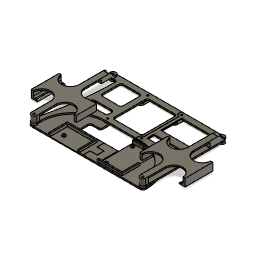
InnerBracket (Autodesk Fusion 360 design; units mm, degrees)
Autodesk Fusion 360 part; units mm, degrees
note: some values were not read from the file. Set by a fixed rule: which face or edge a step refers to.
(part 1 of 2)
sketch "Sketch1" plane through (0, 0, 0) normal (0, 1, 0) x (1, 0, 0) in component "LeftSide"
  line L0 (0, 0) -> (0, -114)
  circle A0 centre (0, 0) radius 1.35
  circle A1 centre (0, -114) radius 1.35
  circle A2 centre (0, -114) radius 4
  circle A3 centre (0, 0) radius 4
  line L1 (0, 0) -> (0, -4)
  line L2 (0, 0) -> (0, 4)
  line L3 (0, 4) -> (10, 4)
  line L4 (10, 4) -> (0, 4)
  line L5 (0, 4) -> (0, -4)
  line L6 (0, -4) -> (10, -4)
  line L7 (10, -4) -> (10, 4)
  line L8 (0, -110) -> (-4, -110)
  line L9 (0, -114) -> (4, -114)
  line L10 (4, -114) -> (-4, -114)
  line L11 (-4, -114) -> (-4, -110)
  line L12 (-4, -110) -> (4, -110)
  line L13 (4, -110) -> (4, -114)
  arc A4 (-4, -110) -> (10, -4) centre (-398.2857, -4) ccw
  line L14 (0, 0) -> (50, 0)
  circle A5 centre (50, 0) radius 1.35
  line L15 (50, 0) -> (99, 0)
  circle A6 centre (99, 0) radius 1.35
  line L16 (99, 0) -> (99, -58)
  line L17 (50, 0) -> (50, -58)
  line L18 (50, -58) -> (99, -58)
  circle A7 centre (99, -58) radius 1.35
  circle A8 centre (50, -58) radius 1.35
  circle A9 centre (50, -58) radius 4
  circle A10 centre (99, -58) radius 4
  circle A11 centre (99, 0) radius 4
  circle A12 centre (50, 0) radius 4
  line L19 (103, 0) -> (103, -58)
  line L20 (99, -62) -> (50, -62)
  line L21 (99, 4) -> (50, 4)
  line L22 (50, 4) -> (10, 4)
  arc A13 (50, -62) -> (4, -110) centre (50, -108.0417) ccw
  dimension "d1" = 114
  dimension "d2" = 2.7
  dimension "d3" = 2.7
  dimension "d4" = 8
  dimension "d5" = 8
  dimension "d6" = 10
  dimension "d7" = 4
  dimension "d8" = 50
  dimension "d9" = 2.7
  dimension "d10" = 49
  dimension "d11" = 2.7
  dimension "d12" = 58
  dimension "d13" = 58
  dimension "d14" = 2.7
  dimension "d15" = 2.7
  dimension "d16" = 8
  dimension "d17" = 8
  dimension "d18" = 8
  dimension "d19" = 8
  constraint coincident L0.start A0.centre
  constraint vertical L0
  constraint coincident L0.end A1.centre
  constraint concentric A1 A2
  constraint concentric A0 A3
  constraint coincident L0 L1.end
  constraint coincident A3 L1.end
  constraint coincident A3 L2.end
  constraint parallel L1 L2
  constraint perpendicular L2 L3
  constraint horizontal L4
  constraint vertical L5
  constraint horizontal L6
  constraint vertical L7
  constraint coincident A2 L8.start
  constraint coincident L0 L8.start
  constraint perpendicular L0 L8
  constraint coincident A2 L9.end
  constraint perpendicular L0 L9
  constraint horizontal L10
  constraint vertical L11
  constraint horizontal L12
  constraint vertical L13
  constraint tangent L7 A4
  constraint perpendicular L0 L14
  constraint coincident L14.end A5.centre
  constraint parallel L14 L15
  constraint coincident L15.end A6.centre
  constraint perpendicular L15 L16
  constraint perpendicular L14 L17
  constraint coincident L16.end L18.end
  constraint coincident L17.end L18.start
  constraint concentric A8 A9
  constraint concentric A7 A10
  constraint concentric A6 A11
  constraint concentric A5 A12
  constraint coincident A11 L19.start
  constraint coincident A10 L19.end
  constraint tangent A10 L19
  constraint vertical L19
  constraint coincident A10 L20.start
  constraint coincident A9 L20.end
  constraint tangent A9 L20
  constraint perpendicular L19 L20
  constraint coincident A11 L21.start
  constraint coincident A12 L21.end
  constraint tangent A12 L21
  constraint parallel L20 L21
  constraint tangent A9 A13
  measures "d1" distance of L0.start L0.end
  measures "d2" diameter of A0
  measures "d3" diameter of A1
  measures "d4" diameter of A2
  measures "d5" diameter of A3
  measures "d6" distance of L2.end L3.end
  measures "d7" distance of L8.start L8.end
  measures "d8" distance of L0.start L14.end
  measures "d9" diameter of A5
  measures "d10" distance of L14.end L15.end
  measures "d11" diameter of A6
  measures "d12" distance of L15.end L16.end
  measures "d13" distance of L14.end L17.end
  measures "d14" diameter of A7
  measures "d15" diameter of A8
  measures "d16" diameter of A9
  measures "d17" diameter of A10
  measures "d18" diameter of A11
  measures "d19" diameter of A12
extrude "Extrude1" add sketch "Sketch1" along normal blind 2 contours L0 A0 A3 L1 L5 L14 | L0 A0 A3 L1 L2 L5 | A0 A3 L2 L5 L14 | A3 L6 L7 L14 | A3 L3 L4 L7 L14 | L0 L7 L12 A4 L14 L17 A9 A12 A13 | L0 L8 L12 A4 | L7 L14 A12 L22 | L0 A1 A2 L9 L10 | A2 L12 L13 | L0 A1 A2 L10 | A2 L8 L11 L12 | L15 A11 A12 L21 | L14 A5 L15 A12 | L14 A5 L17 A12 | A1 A2 L9 L10 | A5 L15 L17 A12 | L15 L16 L17 L18 A9 A10 A11 A12 | L15 A6 L16 A11 | L17 L18 A8 A9 | L18 A9 A10 L20 | L15 A6 L16 A11 | L16 A10 A11 L19 | L17 L18 A8 A9 | L16 L18 A7 A10 | L16 L18 A7 A10 makes body 1 in component "LeftSide"
sketch "Sketch2" plane through (0, 0, 0) normal (0, -1, 0) x (1, 0, 0) in component "LeftSide"
  circle A0 centre (99, 58) radius 1.35
  circle A1 centre (50, 0) radius 1.35
  circle A2 centre (0, 0) radius 1.35
  circle A3 centre (0, 114) radius 1.35
  circle A4 centre (50, 58) radius 1.35
  circle A5 centre (99, 0) radius 1.35
  arc A6 (103, 58) -> (99, 62) centre (99, 58) ccw
  line L0 (99, 62) -> (50, 62)
  arc A7 (4, 110) -> (50, 62) centre (50, 108.0417) ccw
  line L1 (4, 110) -> (4, 114)
  arc A8 (4, 114) -> (-4, 114) centre (0, 114) ccw
  line L2 (-4, 114) -> (-4, 110)
  arc A9 (10, 4) -> (-4, 110) centre (-398.2857, 4) ccw
  line L3 (10, 4) -> (0, 4)
  arc A10 (0, 4) -> (0, -4) centre (0, 0) ccw
  line L4 (0, -4) -> (99, -4)
  arc A11 (99, -4) -> (103, 0) centre (99, 0) ccw
  line L5 (103, 0) -> (103, 58)
  circle A12 centre (0, 0) radius 4
  circle A13 centre (0, 114) radius 4
  circle A14 centre (99, 58) radius 4
  circle A15 centre (50, 58) radius 4
  circle A16 centre (50, 0) radius 4
  circle A17 centre (99, 0) radius 4
  line L6 (50, 0) -> (50, 10)
  line L7 (99, 0) -> (99, 10)
  circle A18 centre (99, 10) radius 4
  circle A19 centre (50, 10) radius 4
  line L8 (95, 10) -> (95, 0)
  line L9 (54, 10) -> (54, 0)
  line L10 (46, 10) -> (46, 0)
  dimension "d404" = 10
  dimension "d405" = 10
  dimension "d406" = 8
  dimension "d407" = 8
  constraint concentric A2 A12
  constraint coincident L3.end A12
  constraint concentric A3 A13
  constraint concentric A0 A14
  constraint coincident A6.end A14
  constraint concentric A4 A15
  constraint coincident L0.end A15
  constraint concentric A1 A16
  constraint tangent L4 A16
  constraint concentric A5 A17
  constraint coincident L4.end A17
  constraint coincident A1.centre A16.centre
  constraint perpendicular L4 L6
  constraint coincident A5.centre A11.centre
  constraint vertical L7
  constraint coincident L7.end A18.centre
  constraint coincident L6.end A19.centre
  constraint coincident A18 L8.start
  constraint coincident A17 L8.end
  constraint tangent A17 L8
  constraint parallel L7 L8
  constraint coincident A19 L9.start
  constraint coincident A16 L9.end
  constraint tangent A16 L9
  constraint parallel L6 L9
  constraint coincident A19 L10.start
  constraint coincident A16 L10.end
  constraint tangent A16 L10
  constraint parallel L6 L10
  measures "d404" distance of A1.centre L6.end
  measures "d405" distance of A5.centre L7.end
  measures "d406" diameter of A18
  measures "d407" diameter of A19
extrude "Extrude2" add sketch "Sketch2" along normal blind 3 contours A6 A14 | A15 | A16 | A18 | L5 A17 L7 A18 | A11 A17 | A17 L7 A18 L8 | A8 A13 | A10 A12 | A16 L6 A19 L10 | A16 L6 A19 L9 | A19 bodies 1 in component "LeftSide"
sketch "Sketch3" plane through (0, 2, 0) normal (0, 1, 0) x (-1, 0, 0) in component "LeftSide"
  circle A0 centre (-99, 58) radius 1.35
  circle A1 centre (-50, 0) radius 1.35
  circle A2 centre (0, 0) radius 1.35
  circle A3 centre (0, 114) radius 1.35
  circle A4 centre (-50, 58) radius 1.35
  circle A5 centre (-99, 0) radius 1.35
  arc A6 (-99, 62) -> (-103, 58) centre (-99, 58) ccw
  line L0 (-103, 58) -> (-103, 0)
  arc A7 (-103, 0) -> (-99, -4) centre (-99, 0) ccw
  line L1 (-99, -4) -> (0, -4)
  arc A8 (0, -4) -> (0, 4) centre (0, 0) ccw
  line L2 (0, 4) -> (-10, 4)
  arc A9 (4, 110) -> (-10, 4) centre (398.2857, 4) ccw
  line L3 (4, 110) -> (4, 114)
  arc A10 (4, 114) -> (-4, 114) centre (0, 114) ccw
  line L4 (-4, 114) -> (-4, 110)
  arc A11 (-50, 62) -> (-4, 110) centre (-50, 108.0417) ccw
  line L5 (-50, 62) -> (-99, 62)
  circle A12 centre (-99, 0) radius 4
  circle A13 centre (-99, 58) radius 4
  line L6 (-95, 58) -> (-95, 62)
  line L7 (-99, 54) -> (-103, 54)
  line L8 (-99, 4) -> (-103, 4)
  line L9 (-95, 0) -> (-95, -4)
  line L10 (-99, 54) -> (-99, 4)
  constraint concentric A5 A12
  constraint coincident A7.end A12
  constraint concentric A0 A13
  constraint coincident A6.start A13
  constraint coincident A13 L6.start
  constraint coincident L5 L6.end
  constraint tangent A13 L6
  constraint perpendicular L5 L6
  constraint coincident A13 L7.start
  constraint coincident L0 L7.end
  constraint tangent A13 L7
  constraint perpendicular L0 L7
  constraint coincident A12 L8.start
  constraint coincident L0 L8.end
  constraint tangent A12 L8
  constraint perpendicular L0 L8
  constraint coincident A12 L9.start
  constraint coincident L1 L9.end
  constraint tangent A12 L9
  constraint perpendicular L1 L9
extrude "Extrude3" cut sketch "Sketch3" against normal blind 1 contours A6 A13 | L5 A13 L6 | L0 A13 L7 | L0 L7 L8 L10 | L0 A12 L8 | A7 A12 | L1 A12 L9 bodies 1 in component "LeftSide"
sketch "Sketch1 (2)" plane through (0, 1, 0) normal (0, 1, 0) x (-1, 0, 0) in component "RightSide"
  circle A0 centre (-99, 58) radius 1.35
  circle A1 centre (-99, 0) radius 1.35
  line L0 (-95, 58) -> (-95, 62)
  line L1 (-95, 62) -> (-99, 62)
  arc A2 (-99, 62) -> (-103, 58) centre (-99, 58) ccw
  line L2 (-103, 58) -> (-103, 0)
  arc A3 (-103, 0) -> (-99, -4) centre (-99, 0) ccw
  line L3 (-99, -4) -> (-95, -4)
  line L4 (-95, -4) -> (-95, 0)
  arc A4 (-95, 0) -> (-99, 4) centre (-99, 0) ccw
  line L5 (-99, 4) -> (-99, 54)
  arc A5 (-99, 54) -> (-95, 58) centre (-99, 58) ccw
  line L6 (-99, 0) -> (-157, 0)
  circle A6 centre (-157, 0) radius 1.35
  circle A7 centre (-157, 0) radius 4
  line L7 (-157, 0) -> (-157, 114)
  circle A8 centre (-157, 114) radius 1.35
  circle A9 centre (-157, 114) radius 4
  line L8 (-161, 114) -> (-161, 0)
  line L9 (-157, -4) -> (-99, -4)
  arc A10 (-153, 114) -> (-99, 62) centre (-100.963, 114) ccw
  dimension "d30" = 58
  dimension "d31" = 2.7
  dimension "d32" = 8
  dimension "d33" = 114
  dimension "d34" = 2.7
  dimension "d35" = 8
  constraint coincident A1.centre A3.centre
  constraint perpendicular L2 L6
  constraint coincident L6.end A6.centre
  constraint concentric A6 A7
  constraint perpendicular L6 L7
  constraint coincident L7.end A8.centre
  constraint concentric A8 A9
  constraint coincident A9 L8.start
  constraint coincident A7 L8.end
  constraint tangent A7 L8
  constraint vertical L8
  constraint coincident A7 L9.start
  constraint coincident A3.end L3.start
  constraint tangent A9 A10
  constraint coincident A9 A10.start
  constraint coincident L1.end A2.start
  measures "d30" distance of A1.centre L6.end
  measures "d31" diameter of A6
  measures "d32" diameter of A7
  measures "d33" distance of L6.end L7.end
  measures "d34" diameter of A8
  measures "d35" diameter of A9
extrude "Extrude1'" add sketch "Sketch1 (2)" along normal blind 1 separate body contours L0 L1 A2 L2 A3 L3 L4 A4 L5 A5 A10 | A2 L2 L6 A7 L7 A9 A10 | A9 | A3 L6 A7 L9 | A7 L7 A9 L8 | L6 A6 A7 L7 | L6 A6 A7 L7 makes body 2 in component "RightSide"
extrude "Extrude2'" add sketch "Sketch1 (2)" against normal blind 1 contours A2 L2 L6 A7 L7 A9 A10 | A9 | A3 L6 A7 L9 | A7 L7 A9 L8 | L6 A6 A7 L7 | L6 A6 A7 L7 bodies 2 in component "RightSide"
sketch "Sketch2 (2)" plane through (0, 0, 0) normal (0, -1, 0) x (1, 0, 0) in component "RightSide"
  circle A0 centre (157, 0) radius 1.35
  circle A1 centre (157, 114) radius 1.35
  line L0 (161, 0) -> (161, 114)
  arc A2 (161, 114) -> (153, 114) centre (157, 114) ccw
  arc A3 (99.2801, 61.9902) -> (153, 114) centre (100.963, 114) ccw
  arc A4 (103, 58) -> (99.2801, 61.9902) centre (99, 58) ccw
  line L1 (103, 58) -> (103, 0)
  arc A5 (99, -4) -> (103, 0) centre (99, 0) ccw
  line L2 (99, -4) -> (157, -4)
  arc A6 (157, -4) -> (161, 0) centre (157, 0) ccw
  circle A7 centre (157, 0) radius 4
  circle A8 centre (157, 114) radius 4
  constraint concentric A0 A7
  constraint coincident L2.end A7
  constraint concentric A1 A8
extrude "Extrude3'" add sketch "Sketch2 (2)" along normal blind 3 contours A6 A7 | A2 A8 bodies 2 in component "RightSide"
sketch "Sketch5" plane through (0, 2, 0) normal (0, 1, 0) x (-1, 0, 0) in component "LeftSide"
  line L0 (-95, 62) -> (-95, 58)
  arc A0 (-99, 54) -> (-95, 58) centre (-99, 58) ccw
  line L1 (-99, 54) -> (-99, 4)
  arc A1 (-95, 0) -> (-99, 4) centre (-99, 0) ccw
  line L2 (-95, 0) -> (-95, -4)
  line L3 (-95, -4) -> (0, -4)
  arc A2 (0, -4) -> (0, 4) centre (0, 0) ccw
  line L4 (0, 4) -> (-10, 4)
  arc A3 (4, 110) -> (-10, 4) centre (398.2857, 4) ccw
  line L5 (4, 110) -> (4, 114)
  arc A4 (4, 114) -> (-4, 114) centre (0, 114) ccw
  line L6 (-4, 114) -> (-4, 110)
  arc A5 (-50, 62) -> (-4, 110) centre (-50, 108.0417) ccw
  line L7 (-50, 62) -> (-95, 62)
  circle A6 centre (0, 114) radius 1.35
  circle A7 centre (0, 0) radius 1.35
  line L8 (-50, 0) -> (-99, 58)
  line L9 (-99, 58) -> (-95.7732, 54.1806)
  line L10 (-50, 0) -> (-53.2268, 3.8194)
  line L11 (-53.2268, 3.8194) -> (-95.7732, 3.8194)
  line L12 (-95.7732, 3.8194) -> (-95.7732, 54.1806)
  line L13 (-95.7732, 54.1806) -> (-53.2268, 54.1806)
  line L14 (-53.2268, 54.1806) -> (-53.2268, 3.8194)
  line L15 (-53.2268, 3.8194) -> (-45.2268, 3.8194)
  line L16 (-45.2268, 3.8194) -> (-15.2268, 3.8194)
  line L17 (-15.2268, 3.8194) -> (-15.2268, 33.8194)
  line L18 (-15.2268, 33.8194) -> (-45.2268, 33.8194)
  line L19 (-45.2268, 33.8194) -> (-45.2268, 3.8194)
  line L20 (-53.2268, 54.1806) -> (-45.2268, 54.1806)
  line L21 (-45.2268, 54.1806) -> (-15.2268, 54.1806)
  line L22 (-15.2268, 54.1806) -> (-15.2268, 44.1806)
  line L23 (-15.2268, 44.1806) -> (-45.2268, 44.1806)
  line L24 (-45.2268, 44.1806) -> (-45.2268, 54.1806)
  circle A8 centre (-50, 58) radius 1.35
  circle A9 centre (-50, 0) radius 1.35
  dimension "d54" = 5
  dimension "d55" = 5
  dimension "d56" = 8
  dimension "d57" = 30
  dimension "d58" = 30
  dimension "d59" = 8
  dimension "d60" = 30
  dimension "d61" = 10
  constraint coincident A0.centre L8.end
  constraint parallel L8 L9
  constraint parallel L8 L10
  constraint horizontal L11
  constraint vertical L12
  constraint horizontal L13
  constraint vertical L14
  constraint perpendicular L14 L15
  constraint horizontal L16
  constraint vertical L17
  constraint horizontal L18
  constraint vertical L19
  constraint perpendicular L14 L20
  constraint horizontal L21
  constraint vertical L22
  constraint horizontal L23
  constraint vertical L24
  measures "d54" distance of A0.centre L9.end
  measures "d55" distance of L8.start L10.end
  measures "d56" distance of L10.end L15.end
  measures "d57" distance of L15.end L16.end
  measures "d58" distance of L15.end L18.end
  measures "d59" distance of L13.end L20.end
  measures "d60" distance of L20.end L21.end
  measures "d61" distance of L20.end L23.end
extrude "Extrude5" cut sketch "Sketch5" against normal blind 2 contours L8 L11 L12 | L8 L13 L14 | L16 L17 L18 L19 | L21 L22 L23 L24 bodies 1 in component "LeftSide"
sketch "Sketch4" plane through (0, 2, 0) normal (0, 1, 0) x (-1, 0, 0) in component "RightSide"
  circle A0 centre (-157, 0) radius 1.35
  circle A1 centre (-157, 114) radius 1.35
  line L0 (-161, 114) -> (-161, 0)
  arc A2 (-161, 0) -> (-157, -4) centre (-157, 0) ccw
  line L1 (-157, -4) -> (-95, -4)
  line L2 (-95, -4) -> (-95, 0)
  arc A3 (-95, 0) -> (-99, 4) centre (-99, 0) ccw
  line L3 (-99, 4) -> (-99, 54)
  arc A4 (-99, 54) -> (-95, 58) centre (-99, 58) ccw
  line L4 (-95, 58) -> (-95, 62)
  line L5 (-95, 62) -> (-99, 62)
  arc A5 (-153, 114) -> (-99, 62) centre (-100.963, 114) ccw
  arc A6 (-153, 114) -> (-161, 114) centre (-157, 114) ccw
  line L6 (-99, 4) -> (-103, 4)
  line L7 (-103, 4) -> (-153, 4)
  line L8 (-153, 4) -> (-153, 34)
  line L9 (-153, 34) -> (-103, 34)
  line L10 (-103, 34) -> (-103, 4)
  line L11 (-99, 54) -> (-103, 54)
  line L12 (-103, 54) -> (-153, 54)
  line L13 (-153, 54) -> (-153, 44)
  line L14 (-153, 44) -> (-103, 44)
  line L15 (-103, 44) -> (-103, 54)
  line L16 (-153, 54) -> (-153, 62)
  line L17 (-153, 62) -> (-152.0608, 62)
  line L18 (-152.0608, 62) -> (-122.0608, 62)
  line L19 (-153, 62) -> (-153, 92)
  arc A7 (-153, 92) -> (-122.0608, 62) centre (-122.9857, 92) ccw
  circle A8 centre (-99, 0) radius 1.35
  circle A9 centre (-99, 58) radius 1.35
  dimension "d64" = 4
  dimension "d65" = 50
  dimension "d66" = 30
  dimension "d67" = 4
  dimension "d68" = 50
  dimension "d69" = 10
  dimension "d105" = 8
  dimension "d106" = 30
  dimension "d107" = 30
  constraint coincident A3.end L3.start
  constraint perpendicular L3 L6
  constraint horizontal L7
  constraint vertical L8
  constraint horizontal L9
  constraint vertical L10
  constraint coincident L3.end A4.start
  constraint perpendicular L3 L11
  constraint horizontal L12
  constraint vertical L13
  constraint horizontal L14
  constraint vertical L15
  constraint perpendicular L12 L16
  constraint perpendicular L16 L17
  constraint perpendicular L16 L18
  constraint perpendicular L17 L19
  constraint tangent L19 A7
  measures "d64" distance of A3.end L6.end
  measures "d65" distance of L6.end L7.end
  measures "d66" distance of L6.end L9.end
  measures "d67" distance of L3.end L11.end
  measures "d68" distance of L11.end L12.end
  measures "d69" distance of L11.end L14.end
  measures "d105" distance of L12.end L16.end
  measures "d106" distance of L17.end L18.end
  measures "d107" distance of L16.end L19.end
extrude "Extrude5'" cut sketch "Sketch4" against normal blind 2 contours L7 L8 L9 L10 | L12 L13 L14 L15 | L17 L18 L19 A7 bodies 2 in component "RightSide"
fillet "Fillet3" radius 3 13 edges at (15.2268, 1, 3.8194) (45.2268, 1, 3.8194) (10, 1, 4) (45.2268, 1, 33.8194) (15.2268, 1, 33.8194) (15.2268, 1, 54.1806) (45.2268, 1, 54.1806) (45.2268, 1, 44.1806) (15.2268, 1, 44.1806) (53.2268, 1, 3.8194) (53.2268, 1, 54.1806) (95.7732, 1, 54.1806) (95.7732, 1, 3.8194) on bodies 1 in component "LeftSide"
fillet "Fillet3'" radius 3 5 edges at (153, 1, 4) (153, 1, 34) (153, 1, 54) (153, 1, 44) (153, 1, 62) on bodies 2 in component "RightSide"
fillet "Fillet4" radius 1 2 edges at (123.9107, 1, 62) (153, 1, 92) on bodies 2 in component "RightSide"
move_face "OffsetFaces1" offset -0.2 5 faces at (98.8097, 1.3333, 3.9955) (95, 1.6667, -1.3333) (99, 1.3333, 37.3333) (98.8097, 1.6667, 54.0045) (95, 1.6667, 59.3333) on bodies 1 in component "LeftSide"
sketch "Sketch1 (3)" plane through (0, 2, 0) normal (0, 1, 0) x (-1, 0, 0) in component "LeftBatteryMount"
  line L0 (-18.2268, 3.8194) -> (-42.2268, 3.8194)
  arc A0 (-45.2268, 6.8194) -> (-42.2268, 3.8194) centre (-42.2268, 6.8194) ccw
  line L1 (-45.2268, 6.8194) -> (-45.2268, 30.8194)
  arc A1 (-42.2268, 33.8194) -> (-45.2268, 30.8194) centre (-42.2268, 30.8194) ccw
  line L2 (-42.2268, 33.8194) -> (-18.2268, 33.8194)
  arc A2 (-15.2268, 30.8194) -> (-18.2268, 33.8194) centre (-18.2268, 30.8194) ccw
  line L3 (-15.2268, 30.8194) -> (-15.2268, 6.8194)
  arc A3 (-18.2268, 3.8194) -> (-15.2268, 6.8194) centre (-18.2268, 6.8194) ccw
  line L4 (-15.2268, 51.1806) -> (-15.2268, 47.1806)
  arc A4 (-18.2268, 44.1806) -> (-15.2268, 47.1806) centre (-18.2268, 47.1806) ccw
  line L5 (-18.2268, 44.1806) -> (-42.2268, 44.1806)
  arc A5 (-45.2268, 47.1806) -> (-42.2268, 44.1806) centre (-42.2268, 47.1806) ccw
  line L6 (-45.2268, 47.1806) -> (-45.2268, 51.1806)
  arc A6 (-42.2268, 54.1806) -> (-45.2268, 51.1806) centre (-42.2268, 51.1806) ccw
  line L7 (-42.2268, 54.1806) -> (-18.2268, 54.1806)
  arc A7 (-15.2268, 51.1806) -> (-18.2268, 54.1806) centre (-18.2268, 51.1806) ccw
  line L8 (-95.7732, 6.8194) -> (-95.7732, 51.1806)
  arc A8 (-92.7732, 54.1806) -> (-95.7732, 51.1806) centre (-92.7732, 51.1806) ccw
  line L9 (-92.7732, 54.1806) -> (-56.2268, 54.1806)
  arc A9 (-53.2268, 51.1806) -> (-56.2268, 54.1806) centre (-56.2268, 51.1806) ccw
  line L10 (-53.2268, 51.1806) -> (-53.2268, 6.8194)
  arc A10 (-56.2268, 3.8194) -> (-53.2268, 6.8194) centre (-56.2268, 6.8194) ccw
  line L11 (-56.2268, 3.8194) -> (-92.7732, 3.8194)
  arc A11 (-95.7732, 6.8194) -> (-92.7732, 3.8194) centre (-92.7732, 6.8194) ccw
  line L12 (-94.8, 62) -> (-94.8, 58)
  arc A12 (-98.8, 53.8048) -> (-94.8, 58) centre (-99, 58) ccw
  line L13 (-98.8, 53.8048) -> (-98.8, 4.1952)
  arc A13 (-94.8, 0) -> (-98.8, 4.1952) centre (-99, 0) ccw
  line L14 (-94.8, 0) -> (-94.8, -4)
  line L15 (-94.8, -4) -> (0, -4)
  arc A14 (0, -4) -> (0, 4) centre (0, 0) ccw
  line L16 (0, 4) -> (-6.9889, 4)
  arc A15 (-9.9888, 7.0222) -> (-6.9889, 4) centre (-6.9889, 7) ccw
  arc A16 (4, 110) -> (-9.9888, 7.0222) centre (398.2857, 4) ccw
  line L17 (4, 110) -> (4, 114)
  arc A17 (4, 114) -> (-4, 114) centre (0, 114) ccw
  line L18 (-4, 114) -> (-4, 110)
  arc A18 (-50, 62) -> (-4, 110) centre (-50, 108.0417) ccw
  line L19 (-50, 62) -> (-94.8, 62)
  circle A19 centre (-50, 58) radius 1.35
  circle A20 centre (0, 114) radius 1.35
  circle A21 centre (0, 0) radius 1.35
  circle A22 centre (-50, 0) radius 1.35
  circle A23 centre (0, 114) radius 4
  line L20 (0, 110) -> (4, 110)
  line L21 (0, 110) -> (-4, 110)
  circle A24 centre (0, 0) radius 4
  line L22 (-4, 110) -> (-4, 21)
  line L23 (-4, 21) -> (4, 21)
  line L24 (4, 21) -> (4, 0)
  line L25 (4, 0) -> (-4, 0)
  line L26 (-4, 0) -> (-4, 21)
  dimension "d154" = 8
  dimension "d155" = 8
  dimension "d156" = 89
  constraint concentric A17 A23
  constraint coincident A23 L20.start
  constraint coincident A16.start L17.start
  constraint tangent A23 L20
  constraint coincident L18.end A18.end
  constraint concentric A14 A24
  constraint perpendicular L21 L22
  constraint horizontal L23
  constraint vertical L24
  constraint horizontal L25
  constraint vertical L26
  constraint midpoint A14 L24.end
  measures "d154" diameter of A23
  measures "d155" diameter of A24
  measures "d156" distance of L18.end L22.end
extrude "Extrude1''" add sketch "Sketch1 (3)" along normal blind 2 separate body contours L18 A23 L21 | A17 A23 | L17 A23 L20 | A14 L16 A24 L23 L24 L26 | L16 A24 L26 | A14 A21 A24 L25 | A14 A21 A24 L25 makes body 3 at (-0.0336, 2, 110.8846) makes body 4 at (0.0336, 2, 14.4487) in component "LeftBatteryMount"
sketch "Sketch2 (3)" plane through (0, 4, 0) normal (0, 1, 0) x (-1, 0, 0) in component "LeftBatteryMount"
  circle A0 centre (0, 0) radius 1.35
  arc A1 (-4, 0) -> (4, 0) centre (0, 0) ccw
  line L0 (4, 0) -> (4, 21)
  line L1 (4, 21) -> (-4, 21)
  line L2 (-4, 21) -> (-4, 0)
  line L3 (-4, 21) -> (4, 21)
  line L4 (4, 21) -> (4, 5)
  line L5 (4, 5) -> (-4, 5)
  line L6 (-4, 5) -> (-4, 21)
  dimension "d159" = 16
  constraint horizontal L3
  constraint vertical L4
  constraint horizontal L5
  constraint vertical L6
  constraint coincident L1.end L2.start
  measures "d159" distance of L1.end L5.end
extrude "Extrude2''" add sketch "Sketch2 (3)" 1 faces at (-0.0336, 4, 110.8846) along normal blind 5 contours L0 L1 L2 L3 L4 L5 L6 on bodies 3 bodies 3 4 in component "LeftBatteryMount"
sketch "Sketch3 (2)" plane through (0, 9, 0) normal (0, 1, 0) x (-1, 0, 0) in component "LeftBatteryMount"
  line L0 (-4, 5) -> (4, 5)
  line L1 (4, 5) -> (4, 21)
  line L2 (4, 21) -> (-4, 21)
  line L3 (-4, 21) -> (-4, 5)
  line L4 (-4, 21) -> (4, 21)
  line L5 (4, 21) -> (4, 110)
  line L6 (4, 110) -> (-4, 110)
  line L7 (-4, 110) -> (-4, 21)
  dimension "d162" = 8
  dimension "d163" = 89
  constraint horizontal L4
  constraint vertical L5
  constraint horizontal L6
  constraint vertical L7
  constraint coincident L2.end L3.start
  measures "d162" distance of L2.end L1.end
  measures "d163" distance of L2.end L6.end
extrude "Extrude3''" add sketch "Sketch3 (2)" 1 faces at (-0.0336, 9, 110.8846) along normal blind 2 on bodies 3 bodies 3 4 in component "LeftBatteryMount"
sketch "Sketch4 (2)" plane through (0, 9, 0) normal (0, -1, 0) x (1, 0, 0) in component "LeftBatteryMount"
  line L0 (4, 110) -> (-4, 110)
  line L1 (-4, 110) -> (-4, 21)
  line L2 (-4, 21) -> (4, 21)
  line L3 (4, 21) -> (4, 110)
  line L4 (-4, 65.5) -> (-29.5, 65.5)
  line L5 (4, 65.5) -> (29.5, 65.5)
  line L6 (-29.5, 65.5) -> (-29.5, 85.5)
  line L7 (-29.5, 85.5) -> (-32.5, 85.5)
  line L8 (-32.5, 85.5) -> (-32.5, 45.5)
  line L9 (-32.5, 45.5) -> (-29.5, 45.5)
  line L10 (-29.5, 45.5) -> (-29.5, 85.5)
  line L11 (29.5, 65.5) -> (29.5, 85.5)
  line L12 (29.5, 85.5) -> (32.5, 85.5)
  line L13 (32.5, 85.5) -> (32.5, 45.5)
  line L14 (32.5, 45.5) -> (29.5, 45.5)
  line L15 (29.5, 45.5) -> (29.5, 85.5)
  line L16 (-16.75, 65.5) -> (-16.75, 73.5)
  line L17 (-16.75, 65.5) -> (-16.75, 57.5)
  line L18 (16.75, 65.5) -> (16.75, 73.5)
  line L19 (16.75, 65.5) -> (16.75, 57.5)
  arc A0 (-29.5, 85.5) -> (-4, 85.2119) centre (-16.7395, 86.2846) ccw
  arc A1 (-4, 45.5) -> (-29.5, 45.5) centre (-16.75, 44.7266) ccw
  arc A2 (29.5, 45.5) -> (4, 45.5) centre (16.75, 44.7266) ccw
  arc A3 (4, 85.5) -> (29.5, 85.5) centre (16.75, 86.2734) ccw
  dimension "d166" = 25.5
  dimension "d167" = 25.5
  dimension "d168" = 20
  dimension "d169" = 3
  dimension "d170" = 40
  dimension "d171" = 20
  dimension "d172" = 3
  dimension "d173" = 40
  dimension "d174" = 8
  dimension "d175" = 8
  dimension "d176" = 8
  dimension "d177" = 8
  constraint midpoint L1 L4.start
  constraint perpendicular L1 L4
  constraint midpoint L3 L5.start
  constraint perpendicular L3 L5
  constraint perpendicular L4 L6
  constraint horizontal L7
  constraint vertical L8
  constraint horizontal L9
  constraint vertical L10
  constraint perpendicular L5 L11
  constraint horizontal L12
  constraint vertical L13
  constraint horizontal L14
  constraint vertical L15
  constraint midpoint L4 L16.start
  constraint perpendicular L4 L16
  constraint perpendicular L4 L17
  constraint midpoint L5 L18.start
  constraint perpendicular L5 L18
  constraint perpendicular L5 L19
  constraint coincident L16.end A0
  constraint coincident L1 A0.end
  constraint coincident L17.end A1
  constraint coincident L1 A1.start
  constraint coincident L19.end A2
  constraint coincident L3 A2.end
  constraint coincident L18.end A3
  constraint coincident L3 A3.start
  measures "d166" distance of L4.start L4.end
  measures "d167" distance of L5.start L5.end
  measures "d168" distance of L4.end L6.end
  measures "d169" distance of L6.end L7.end
  measures "d170" distance of L6.end L9.end
  measures "d171" distance of L5.end L11.end
  measures "d172" distance of L11.end L12.end
  measures "d173" distance of L11.end L14.end
  measures "d174" distance of L16.start L16.end
  measures "d175" distance of L16.start L17.end
  measures "d176" distance of L18.start L18.end
  measures "d177" distance of L18.start L19.end
extrude "Extrude4" add sketch "Sketch4 (2)" against normal blind 2 contours L3 L5 L18 A3 | L1 L4 L16 A0 | L3 L5 L19 A2 | L5 L11 L15 L18 A3 | L1 L4 L17 A1 | L4 L6 L10 L16 A0 | L5 L15 L19 A2 | L11 L12 L13 L14 L15 | L4 L10 L17 A1 | L6 L7 L8 L9 L10 bodies 3 in component "LeftBatteryMount"
sketch "Sketch5 (2)" plane through (0, 9, 0) normal (0, -1, 0) x (1, 0, 0) in component "LeftBatteryMount"
  line L0 (4, 110) -> (-4, 110)
  line L1 (-4, 110) -> (-4, 85.2119)
  arc A0 (-29.5, 85.5) -> (-4, 85.2119) centre (-16.7395, 86.2846) ccw
  line L2 (-29.5, 85.5) -> (-32.5, 85.5)
  line L3 (-32.5, 85.5) -> (-32.5, 45.5)
  line L4 (-32.5, 45.5) -> (-29.5, 45.5)
  arc A1 (-4, 45.5) -> (-29.5, 45.5) centre (-16.75, 44.7266) ccw
  line L5 (-4, 45.5) -> (-4, 21)
  line L6 (-4, 21) -> (4, 21)
  line L7 (4, 21) -> (4, 45.5)
  arc A2 (29.5, 45.5) -> (4, 45.5) centre (16.75, 44.7266) ccw
  line L8 (29.5, 45.5) -> (32.5, 45.5)
  line L9 (32.5, 45.5) -> (32.5, 85.5)
  line L10 (32.5, 85.5) -> (29.5, 85.5)
  arc A3 (4, 85.5) -> (29.5, 85.5) centre (16.75, 86.2734) ccw
  line L11 (4, 85.5) -> (4, 110)
  line L12 (-29.5, 85.5) -> (-29.5, 45.5)
  line L13 (29.5, 85.5) -> (29.5, 45.5)
  constraint coincident A0.start L2.start
  constraint coincident L4.end A1.end
  constraint coincident L10.end A3.end
  constraint coincident A2.start L8.start
extrude "Extrude5''" add sketch "Sketch5 (2)" along normal blind 7 contours L8 L9 L10 L13 | L2 L3 L4 L12 bodies 3 in component "LeftBatteryMount"
sketch "Sketch6" plane through (0, 2, 0) normal (0, -1, 0) x (1, 0, 0) in component "LeftBatteryMount"
  line L0 (-32.5, 85.5) -> (-32.5, 45.5)
  line L1 (-32.5, 45.5) -> (-29.5, 45.5)
  line L2 (-29.5, 45.5) -> (-29.5, 85.5)
  line L3 (-29.5, 85.5) -> (-32.5, 85.5)
  line L4 (-29.5, 85.5) -> (-23.5, 85.5)
  line L5 (-23.5, 85.5) -> (-23.5, 45.5)
  line L6 (-23.5, 45.5) -> (-29.5, 45.5)
  line L7 (-29.5, 45.5) -> (-29.5, 85.5)
  dimension "d182" = 6
  dimension "d183" = 40
  constraint horizontal L4
  constraint vertical L5
  constraint horizontal L6
  constraint vertical L7
  constraint coincident L2.end L3.start
  measures "d182" distance of L2.end L4.end
  measures "d183" distance of L2.end L1.end
extrude "Extrude6" add sketch "Sketch6" along normal blind 2 bodies 3 in component "LeftBatteryMount"
fillet "Fillet1" radius 5 2 edges at (0, 11, 5) (0, 4, 5) on bodies 3 in component "LeftBatteryMount"
fillet "Fillet2" radius 2 2 edges at (-29.5, 2, 65.5) (-23.5, 2, 65.5) on bodies 3 in component "LeftBatteryMount"
sketch "Sketch1 (4)" plane through (0, 2, 0) normal (0, 1, 0) x (-1, 0, 0) in component "RightBatteryMount"
  line L0 (-153, 7) -> (-153, 31)
  arc A0 (-150, 34) -> (-153, 31) centre (-150, 31) ccw
  line L1 (-150, 34) -> (-103, 34)
  line L2 (-103, 34) -> (-103, 4)
  line L3 (-103, 4) -> (-150, 4)
  arc A1 (-153, 7) -> (-150, 4) centre (-150, 7) ccw
  line L4 (-150, 54) -> (-103, 54)
  line L5 (-103, 54) -> (-103, 44)
  line L6 (-103, 44) -> (-150, 44)
  arc A2 (-153, 47) -> (-150, 44) centre (-150, 47) ccw
  line L7 (-153, 47) -> (-153, 51)
  arc A3 (-150, 54) -> (-153, 51) centre (-150, 51) ccw
  arc A4 (-151.0645, 81.3962) -> (-133.626, 63.9351) centre (-122.9857, 92) ccw
  arc A5 (-133.9805, 62) -> (-133.626, 63.9351) centre (-133.9805, 63) ccw
  line L8 (-133.9805, 62) -> (-150, 62)
  arc A6 (-153, 65) -> (-150, 62) centre (-150, 65) ccw
  line L9 (-153, 65) -> (-153, 81.0429)
  arc A7 (-151.0645, 81.3962) -> (-153, 81.0429) centre (-152, 81.0429) ccw
  circle A8 centre (-157, 0) radius 1.35
  circle A9 centre (-99, 58) radius 1.35
  circle A10 centre (-157, 114) radius 1.35
  circle A11 centre (-99, 0) radius 1.35
  line L10 (-161, 114) -> (-161, 0)
  arc A12 (-161, 0) -> (-157, -4) centre (-157, 0) ccw
  line L11 (-157, -4) -> (-95, -4)
  line L12 (-95, -4) -> (-95, 0)
  arc A13 (-95, 0) -> (-99, 4) centre (-99, 0) ccw
  line L13 (-99, 4) -> (-99, 54)
  arc A14 (-99, 54) -> (-95, 58) centre (-99, 58) ccw
  line L14 (-95, 58) -> (-95, 62)
  line L15 (-95, 62) -> (-99, 62)
  arc A15 (-153, 114) -> (-99, 62) centre (-100.963, 114) ccw
  arc A16 (-153, 114) -> (-161, 114) centre (-157, 114) ccw
  circle A17 centre (-157, 0) radius 4
  circle A18 centre (-157, 114) radius 4
  line L16 (-157, 114) -> (-157, 110)
  line L17 (-153, 114) -> (-153, 110)
  line L18 (-153, 110) -> (-161, 110)
  line L19 (-161, 110) -> (-161, 21)
  line L20 (-161, 21) -> (-153, 21)
  line L21 (-153, 21) -> (-153, 0)
  line L22 (-153, 0) -> (-161, 0)
  line L23 (-161, 0) -> (-161, 21)
  dimension "d190" = 8
  dimension "d191" = 8
  dimension "d192" = 89
  constraint concentric A8 A17
  constraint concentric A10 A18
  constraint coincident A10.centre A16.centre
  constraint coincident A18 L16.end
  constraint vertical L16
  constraint coincident A15.start A16.start
  constraint tangent A15 L17
  constraint coincident L10 L18.end
  constraint perpendicular L10 L18
  constraint perpendicular L18 L19
  constraint horizontal L20
  constraint vertical L21
  constraint horizontal L22
  constraint vertical L23
  constraint coincident A17 L21.end
  measures "d190" diameter of A17
  measures "d191" diameter of A18
  measures "d192" distance of L18.end L19.end
extrude "Extrude1'''" add sketch "Sketch1 (4)" along normal blind 2 separate body contours L0 L10 A17 L20 L21 L23 | A8 A17 L22 | A8 A12 A17 L22 | L10 A18 L18 | A16 A18 | A18 L17 L18 makes body 5 at (157.0336, 2, 14.4487) makes body 6 at (157.0336, 2, 110.8846) in component "RightBatteryMount"
sketch "Sketch2 (4)" plane through (0, 4, 0) normal (0, 1, 0) x (-1, 0, 0) in component "RightBatteryMount"
  circle A0 centre (-157, 0) radius 1.35
  arc A1 (-161, 0) -> (-153, 0) centre (-157, 0) ccw
  line L0 (-153, 0) -> (-153, 21)
  line L1 (-153, 21) -> (-161, 21)
  line L2 (-161, 21) -> (-161, 0)
  line L3 (-161, 21) -> (-153, 21)
  line L4 (-153, 21) -> (-153, 5)
  line L5 (-153, 5) -> (-161, 5)
  line L6 (-161, 5) -> (-161, 21)
  dimension "d195" = 16
  constraint horizontal L3
  constraint vertical L4
  constraint horizontal L5
  constraint vertical L6
  constraint coincident L1.end L2.start
  measures "d195" distance of L1.end L5.end
extrude "Extrude2'''" add sketch "Sketch2 (4)" 1 faces at (157.0336, 4, 110.8846) along normal blind 5 contours L0 L1 L2 L3 L4 L5 L6 on bodies 6 bodies 6 5 in component "RightBatteryMount"
sketch "Sketch3 (3)" plane through (0, 9, 0) normal (0, 1, 0) x (-1, 0, 0) in component "RightBatteryMount"
  line L0 (-161, 5) -> (-153, 5)
  line L1 (-153, 5) -> (-153, 21)
  line L2 (-153, 21) -> (-161, 21)
  line L3 (-161, 21) -> (-161, 5)
  line L4 (-161, 21) -> (-161, 110)
  line L5 (-161, 110) -> (-153, 110)
  line L6 (-153, 110) -> (-153, 21)
  line L7 (-153, 21) -> (-161, 21)
  line L8 (-161, 21) -> (-161, 110)
  dimension "d198" = 89
  constraint coincident L2.end L3.start
  constraint perpendicular L2 L4
  constraint horizontal L5
  constraint vertical L6
  constraint horizontal L7
  constraint vertical L8
  constraint coincident L1.end L2.start
  measures "d198" distance of L2.end L4.end
extrude "Extrude3'''" add sketch "Sketch3 (3)" 1 faces at (157.0336, 9, 110.8846) along normal blind 2 on bodies 6 bodies 6 5 in component "RightBatteryMount"
sketch "Sketch4 (3)" plane through (0, 9, 0) normal (0, -1, 0) x (1, 0, 0) in component "RightBatteryMount"
  line L0 (161, 110) -> (153, 110)
  line L1 (153, 110) -> (153, 21)
  line L2 (153, 21) -> (161, 21)
  line L3 (161, 21) -> (161, 110)
  line L4 (161, 65.5) -> (186.5, 65.5)
  line L5 (153, 65.5) -> (127.5, 65.5)
  line L6 (127.5, 65.5) -> (127.5, 85.5)
  line L7 (186.5, 65.5) -> (186.5, 85.5)
  line L8 (186.5, 85.5) -> (189.5, 85.5)
  line L9 (189.5, 85.5) -> (189.5, 45.5)
  line L10 (189.5, 45.5) -> (186.5, 45.5)
  line L11 (186.5, 45.5) -> (186.5, 85.5)
  line L12 (127.5, 85.5) -> (124.5, 85.5)
  line L13 (124.5, 85.5) -> (124.5, 45.5)
  line L14 (124.5, 45.5) -> (127.5, 45.5)
  line L15 (127.5, 45.5) -> (127.5, 85.5)
  line L16 (140.25, 65.5) -> (140.25, 57.5)
  line L17 (140.25, 65.5) -> (140.25, 73.5)
  line L18 (173.75, 65.5) -> (173.75, 73.5)
  line L19 (173.75, 65.5) -> (173.75, 57.5)
  arc A0 (127.5, 85.5) -> (153, 85.5) centre (140.25, 86.2734) ccw
  arc A1 (161, 85.5) -> (186.5, 85.5) centre (173.75, 86.2734) ccw
  arc A2 (186.5, 45.5) -> (161, 45.5) centre (173.75, 44.7266) ccw
  arc A3 (153, 45.5) -> (127.5, 45.5) centre (140.25, 44.7266) ccw
  dimension "d201" = 25.5
  dimension "d202" = 25.5
  dimension "d203" = 20
  dimension "d204" = 20
  dimension "d205" = 3
  dimension "d206" = 40
  dimension "d207" = 3
  dimension "d208" = 40
  dimension "d209" = 8
  dimension "d210" = 8
  dimension "d211" = 8
  dimension "d212" = 8
  constraint midpoint L3 L4.start
  constraint perpendicular L3 L4
  constraint midpoint L1 L5.start
  constraint perpendicular L1 L5
  constraint perpendicular L5 L6
  constraint perpendicular L4 L7
  constraint horizontal L8
  constraint vertical L9
  constraint horizontal L10
  constraint vertical L11
  constraint horizontal L12
  constraint vertical L13
  constraint horizontal L14
  constraint vertical L15
  constraint midpoint L5 L16.start
  constraint perpendicular L5 L16
  constraint perpendicular L5 L17
  constraint midpoint L4 L18.start
  constraint perpendicular L4 L18
  constraint perpendicular L4 L19
  constraint coincident L17.end A0
  constraint coincident L1 A0.end
  constraint coincident L18.end A1
  constraint coincident L3 A1.start
  constraint coincident L19.end A2
  constraint coincident L3 A2.end
  constraint coincident L16.end A3
  constraint coincident L1 A3.start
  measures "d201" distance of L4.start L4.end
  measures "d202" distance of L5.start L5.end
  measures "d203" distance of L5.end L6.end
  measures "d204" distance of L4.end L7.end
  measures "d205" distance of L7.end L8.end
  measures "d206" distance of L7.end L10.end
  measures "d207" distance of L6.end L12.end
  measures "d208" distance of L6.end L14.end
  measures "d209" distance of L16.start L16.end
  measures "d210" distance of L16.start L17.end
  measures "d211" distance of L18.start L18.end
  measures "d212" distance of L18.start L19.end
extrude "Extrude4'" add sketch "Sketch4 (3)" against normal blind 2 contours L3 L4 L18 A1 | L1 L5 L17 A0 | L3 L4 L19 A2 | L4 L7 L11 L18 A1 | L1 L5 L16 A3 | L5 L6 L15 L17 A0 | L4 L11 L19 A2 | L7 L8 L9 L10 L11 | L5 L15 L16 A3 | L6 L12 L13 L14 L15 bodies 6 in component "RightBatteryMount"
sketch "Sketch5 (3)" plane through (0, 9, 0) normal (0, -1, 0) x (1, 0, 0) in component "RightBatteryMount"
  line L0 (161, 110) -> (153, 110)
  line L1 (153, 110) -> (153, 85.5)
  arc A0 (127.5, 85.5) -> (153, 85.5) centre (140.25, 86.2734) ccw
  line L2 (127.5, 85.5) -> (124.5, 85.5)
  line L3 (124.5, 85.5) -> (124.5, 45.5)
  line L4 (124.5, 45.5) -> (127.5, 45.5)
  arc A1 (153, 45.5) -> (127.5, 45.5) centre (140.25, 44.7266) ccw
  line L5 (153, 45.5) -> (153, 21)
  line L6 (153, 21) -> (161, 21)
  line L7 (161, 21) -> (161, 45.5)
  arc A2 (186.5, 45.5) -> (161, 45.5) centre (173.75, 44.7266) ccw
  line L8 (186.5, 45.5) -> (189.5, 45.5)
  line L9 (189.5, 45.5) -> (189.5, 85.5)
  line L10 (189.5, 85.5) -> (186.5, 85.5)
  arc A3 (161, 85.5) -> (186.5, 85.5) centre (173.75, 86.2734) ccw
  line L11 (161, 85.5) -> (161, 110)
  line L12 (127.5, 85.5) -> (127.5, 45.5)
  line L13 (186.5, 85.5) -> (186.5, 45.5)
  constraint coincident A0.start L2.start
  constraint coincident L4.end A1.end
  constraint coincident L10.end A3.end
  constraint coincident A2.start L8.start
extrude "Extrude5'''" add sketch "Sketch5 (3)" along normal blind 7 contours L8 L9 L10 L13 | L2 L3 L4 L12 bodies 6 in component "RightBatteryMount"
sketch "Sketch6 (2)" plane through (0, 2, 0) normal (0, -1, 0) x (1, 0, 0) in component "RightBatteryMount"
  line L0 (186.5, 85.5) -> (186.5, 45.5)
  line L1 (186.5, 45.5) -> (189.5, 45.5)
  line L2 (189.5, 45.5) -> (189.5, 85.5)
  line L3 (189.5, 85.5) -> (186.5, 85.5)
  line L4 (186.5, 85.5) -> (180.5, 85.5)
  line L5 (180.5, 85.5) -> (180.5, 45.5)
  line L6 (180.5, 45.5) -> (186.5, 45.5)
  line L7 (186.5, 45.5) -> (186.5, 85.5)
  dimension "d217" = 6
  dimension "d218" = 40
  constraint horizontal L4
  constraint vertical L5
  constraint horizontal L6
  constraint vertical L7
  constraint coincident L0.start L3.end
  measures "d217" distance of L0.start L4.end
  measures "d218" distance of L0.start L0.end
extrude "Extrude6'" add sketch "Sketch6 (2)" along normal blind 2 bodies 6 in component "RightBatteryMount"
fillet "Fillet1'" radius 5 2 edges at (157, 11, 5) (157, 4, 5) on bodies 6 in component "RightBatteryMount"
fillet "Fillet2'" radius 2 2 edges at (186.5, 2, 65.5) (180.5, 2, 65.5) on bodies 6 in component "RightBatteryMount"
sketch "Sketch7" plane through (0, 2, 0) normal (0, -1, 0) x (1, 0, 0) in component "LeftBatteryMount"
  circle A0 centre (0, 0) radius 1.35
  arc A1 (-4, 0) -> (4, 0) centre (0, 0) ccw
  line L0 (4, 0) -> (4, 21)
  line L1 (4, 21) -> (-4, 21)
  line L2 (-4, 21) -> (-4, 0)
  line L3 (4, 21) -> (-4, 21)
  line L4 (-4, 21) -> (-4, 6)
  line L5 (-4, 6) -> (4, 6)
  line L6 (4, 6) -> (4, 21)
  dimension "d225" = 15
  constraint horizontal L3
  constraint vertical L4
  constraint horizontal L5
  constraint vertical L6
  constraint coincident L0.end L1.start
  measures "d225" distance of L0.end L5.end
extrude "Extrude7" cut sketch "Sketch7" against normal blind 2 contours L0 L1 L2 L3 L4 L5 L6 bodies 3 in component "LeftBatteryMount"
sketch "Sketch8" plane through (0, 11, 0) normal (0, 1, 0) x (-1, 0, 0) in component "LeftBatteryMount"
  line L0 (-4, 10) -> (4, 10)
  line L1 (4, 10) -> (4, 45.5)
  arc A0 (29.5, 45.5) -> (4, 45.5) centre (16.75, 44.7266) ccw
  line L2 (29.5, 45.5) -> (32.5, 45.5)
  line L3 (32.5, 45.5) -> (32.5, 85.5)
  line L4 (32.5, 85.5) -> (29.5, 85.5)
  arc A1 (4, 85.2119) -> (29.5, 85.5) centre (16.7395, 86.2846) ccw
  line L5 (4, 85.2119) -> (4, 114)
  arc A2 (4, 114) -> (-4, 114) centre (0, 114) ccw
  line L6 (-4, 114) -> (-4, 85.5)
  arc A3 (-29.5, 85.5) -> (-4, 85.5) centre (-16.75, 86.2734) ccw
  line L7 (-29.5, 85.5) -> (-32.5, 85.5)
  line L8 (-32.5, 85.5) -> (-32.5, 45.5)
  line L9 (-32.5, 45.5) -> (-29.5, 45.5)
  arc A4 (-4, 45.5) -> (-29.5, 45.5) centre (-16.75, 44.7266) ccw
  line L10 (-4, 45.5) -> (-4, 10)
  circle A5 centre (0, 114) radius 1.35
  line L11 (-32.5, 56.5031) -> (-21.6971, 56.5031)
  constraint coincident L8 L11.start
  constraint coincident A4 L11.end
  constraint perpendicular L8 L11
extrude "Extrude8" cut sketch "Sketch8" against normal blind 9 contours L8 L9 A4 L11 bodies 3 in component "LeftBatteryMount"
extrude "Extrude8'" cut 3 faces at (3.1018, -3, 114.1987) (95.8982, -3, 58.1987) (53.0967, -3, 58.2658) along direction (0, 1, 0) blind 2 on bodies 1 bodies 1 in component "LeftSide"
sketch "Sketch1 (5)" plane through (0, -1, 0) normal (0, -1, 0) x (1, 0, 0) in component "LeftBoardHolder"
  circle A0 centre (0, 114) radius 1.35
  circle A1 centre (0, 114) radius 4
  line L0 (0, 114) -> (50, 114)
  line L1 (50, 114) -> (50, 58)
  circle A2 centre (50, 58) radius 4
  line L2 (46, 58) -> (0, 110)
  line L3 (50, 114) -> (75, 114)
  line L4 (75, 114) -> (50.0008, 114)
  line L5 (50.0008, 114) -> (50.0008, 54)
  line L6 (50.0008, 54) -> (75, 54)
  line L7 (75, 54) -> (75, 114)
  line L8 (75, 114) -> (0, 114)
  line L9 (0, 114) -> (0, 118)
  line L10 (0, 118) -> (75, 118)
  line L11 (75, 118) -> (75, 114)
  arc A3 (-3.9996, 113.9403) -> (50.0008, 54) centre (57.2823, 114.8546) ccw
  line L12 (50, 58) -> (55, 58)
  line L13 (55, 58) -> (55, 54)
  line L14 (55, 58) -> (55, 88)
  line L15 (55, 88) -> (75, 88)
  dimension "d294" = 50
  dimension "d295" = 56
  dimension "d296" = 8
  dimension "d297" = 25
  dimension "d361" = 5
  dimension "d362" = 30
  constraint coincident A0.centre A1.centre
  constraint horizontal L0
  constraint perpendicular L0 L1
  constraint coincident L1.end A2.centre
  constraint coincident A2 L2.start
  constraint coincident A1 L2.end
  constraint perpendicular L1 L3
  constraint horizontal L4
  constraint vertical L5
  constraint horizontal L6
  constraint vertical L7
  constraint coincident A2 L5.end
  constraint horizontal L8
  constraint vertical L9
  constraint horizontal L10
  constraint vertical L11
  constraint coincident A1 L9.end
  constraint tangent A1 A3
  constraint coincident A1 A3.start
  constraint perpendicular L5 L12
  constraint coincident L6 L13.end
  constraint perpendicular L6 L13
  constraint perpendicular L12 L14
  constraint coincident L7 L15.end
  constraint perpendicular L7 L15
  measures "d294" distance of A0.centre L0.end
  measures "d295" distance of L0.end L1.end
  measures "d296" diameter of A2
  measures "d297" distance of L0.end L3.end
  measures "d361" distance of L1.end L12.end
  measures "d362" distance of L12.end L14.end
extrude "Extrude1''''" add sketch "Sketch1 (5)" along normal blind 2 separate body contours A0 A1 L0 L8 L9 | A0 A1 L0 L8 L9 | A1 L0 L1 A2 L2 L5 L8 | A1 L0 L3 L4 L8 L10 L11 | A1 A2 L2 A3 | L1 A2 L3 L4 L5 L7 L8 L12 L14 L15 | L1 A2 L5 A3 | L1 A2 L5 L12 | A2 A3 | A2 L5 L12 | A2 L6 L12 L13 makes body 7 in component "LeftBoardHolder"
sketch "Sketch2 (5)" plane through (0, -3, 0) normal (0, -1, 0) x (1, 0, 0) in component "LeftBoardHolder"
  circle A0 centre (0, 114) radius 1.35
  line L0 (54, 58) -> (54, 54)
  arc A1 (48.9911, 54.1293) -> (50.0008, 54) centre (50, 58) ccw
  line L1 (50.0008, 54) -> (55, 54)
  line L2 (75, 88) -> (75, 118)
  arc A2 (0, 118) -> (-3.9996, 113.9403) centre (0, 114) ccw
  line L3 (75, 118) -> (0, 118)
  arc A3 (-3.9996, 113.9403) -> (48.9911, 54.1293) centre (57.2823, 114.8546) ccw
  line L4 (54, 58) -> (34.3943, 58)
  line L5 (55, 54) -> (55, 88)
  line L6 (55, 88) -> (75, 88)
  line L7 (55, 59.6605) -> (30.638, 59.6605)
  constraint coincident A3 L4.end
  constraint perpendicular L0 L4
  constraint coincident L5 L7.start
  constraint coincident A3 L7.end
  constraint perpendicular L5 L7
extrude "Extrude2''''" cut sketch "Sketch2 (5)" against normal blind 1 contours L0 L1 A3 L4 L5 L7 | L0 A1 L1 A3 L4 bodies 7 in component "LeftBoardHolder"
sketch "Sketch3 (4)" plane through (0, -1, 0) normal (0, 1, 0) x (-1, 0, 0) in component "LeftBoardHolder"
  circle A0 centre (0, 114) radius 1.35
  arc A1 (-50.0008, 54) -> (-48.9911, 54.1293) centre (-50, 58) ccw
  arc A2 (3.9996, 113.9403) -> (0, 118) centre (0, 114) ccw
  line L0 (-75, 118) -> (-75, 88)
  line L1 (-55, 54) -> (-50.0008, 54)
  line L2 (0, 118) -> (-75, 118)
  line L3 (0, 118) -> (-27, 118)
  line L4 (-27, 118) -> (-27, 93)
  line L5 (-27, 93) -> (-67, 93)
  line L6 (-67, 93) -> (-67, 118)
  line L7 (-67, 118) -> (-27, 118)
  line L8 (-27, 118) -> (-27, 93)
  line L9 (-67, 93) -> (-69, 93)
  line L10 (-69, 93) -> (-69, 91)
  line L11 (-69, 91) -> (-67, 91)
  line L12 (-67, 91) -> (-67, 93)
  line L13 (-27, 118) -> (-25, 118)
  line L14 (-25, 118) -> (-69, 118)
  line L15 (-69, 118) -> (-69, 91)
  line L16 (-69, 91) -> (-25, 91)
  line L17 (-25, 91) -> (-25, 118)
  arc A3 (-48.9911, 54.1293) -> (3.9996, 113.9403) centre (-57.2823, 114.8546) ccw
  line L18 (-55, 88) -> (-55, 54)
  line L19 (-75, 88) -> (-55, 88)
  dimension "d298" = 27
  dimension "d299" = 25
  dimension "d300" = 40
  dimension "d301" = 2
  dimension "d302" = 2
  dimension "d303" = 2
  constraint coincident A2.end L2.start
  constraint parallel L2 L3
  constraint perpendicular L2 L4
  constraint horizontal L5
  constraint vertical L6
  constraint horizontal L7
  constraint vertical L8
  constraint horizontal L9
  constraint vertical L10
  constraint horizontal L11
  constraint vertical L12
  constraint perpendicular L8 L13
  constraint horizontal L14
  constraint vertical L15
  constraint horizontal L16
  constraint vertical L17
  measures "d298" distance of A2.end L3.end
  measures "d299" distance of L3.end L4.end
  measures "d300" distance of L4.end L5.end
  measures "d301" distance of L5.end L9.end
  measures "d302" distance of L5.end L11.end
  measures "d303" distance of L3.end L13.end
extrude "Extrude3''''" cut sketch "Sketch3 (4)" against normal blind 1 contours L2 L4 L5 L6 L7 L8 L14 bodies 7 in component "LeftBoardHolder"
extrude "Extrude6''" add sketch "Sketch3 (4)" along normal blind 3 contours L2 L3 L4 L5 L8 L12 L13 L14 L16 L17 | L2 L6 L9 L14 L15 | L9 L10 L11 L12 L15 L16 bodies 7 in component "LeftBoardHolder"
sketch "Sketch4 (4)" plane through (0, -2, 0) normal (0, 1, 0) x (-1, 0, 0) in component "LeftBoardHolder"
  line L0 (-27, 118) -> (-36, 118)
  line L1 (-36, 118) -> (-36, 107)
  line L2 (-36, 107) -> (-27, 107)
  line L3 (-27, 107) -> (-27, 118)
  circle A0 centre (-36, 107) radius 0.9
  circle A1 centre (-36, 107) radius 2.5
  line L4 (-27, 118) -> (-67, 118)
  line L5 (-67, 118) -> (-67, 93)
  line L6 (-67, 93) -> (-27, 93)
  line L7 (-27, 93) -> (-27, 118)
  dimension "d250" = 9
  dimension "d251" = 11
  dimension "d252" = 1.8
  dimension "d255" = 5
  constraint horizontal L0
  constraint vertical L1
  constraint horizontal L2
  constraint vertical L3
  constraint coincident L1.end L2.start
  constraint concentric A0 A1
  constraint coincident L0.start L3.end
  measures "d250" distance of L0.end L0.start
  measures "d251" distance of L2.end L0.start
  measures "d252" diameter of A0
  measures "d255" diameter of A1
extrude "Extrude4''" cut sketch "Sketch4 (4)" against normal blind 2 contours L1 L2 A0 | L1 L2 A0 bodies 7 in component "LeftBoardHolder"
extrude "Extrude5''''" add sketch "Sketch4 (4)" along normal blind 1 contours L1 L2 A0 A1 | L1 L2 A0 A1 bodies 7 in component "LeftBoardHolder"
extrude "Extrude7'" cut 1 faces at (160.1018, -3, 114.1987) along direction (0, 1, 0) blind 2 on bodies 2 bodies 2 in component "RightSide"